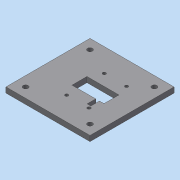
# Autodesk Inventor part: Part2
Saved by Autodesk Inventor 2016 SP1 (Build 200210100, 210)
## iProperties
Created: 2016-03-20
Part Number: Part2
Material: Generic
Document SubType Name: Modeling
Designer: Mohamed A.
Density: 1 g/cm^3
Appearance: Default
Author: Mohamed A.
Autodesk Inventor part; units mm, degrees
ref_plane "YZ Plane" through (0, 0, 0) normal (1, 0, 0) x (0, 1, 0)
ref_plane "XZ Plane" through (0, 0, 0) normal (0, 1, 0) x (-1, 0, 0)
ref_plane "XY Plane" through (0, 0, 0) normal (0, 0, 1) x (1, 0, 0)
sketch "Sketch1" plane through (0, 0, 0) normal (0, 0, 1) x (1, 0, 0)
  line L0 (8.35, -7) -> (8.35, -9) construction
  line L1 (8.35, -9) -> (7.35, -9) construction
  line L2 (7.35, -9) -> (7.35, -7) construction
  line L3 (7.35, -7) -> (8.35, -7) construction
  line L4 (9.45, -5.5) -> (9.45, -7.5) construction
  line L5 (9.45, -7.5) -> (8.45, -7.5) construction
  line L6 (8.45, -7.5) -> (8.45, -5.5) construction
  line L7 (8.45, -5.5) -> (9.45, -5.5) construction
  line L8 (2.45, 4.2) -> (2.45, -4.2) construction
  line L9 (2.45, -4.2) -> (-5.95, -4.2) construction
  line L10 (-5.95, -4.2) -> (-5.95, 4.2) construction
  line L11 (-5.95, 4.2) -> (2.45, 4.2) construction
  circle A0 centre (-2.6, 10.5) radius 1 construction
  circle A1 centre (9.9, 10.5) radius 1 construction
  circle A2 centre (-2.6, -10.5) radius 1 construction
  circle A3 centre (9.9, -10.5) radius 1 construction
  line L12 (11.95, 12.5) -> (-11.95, 12.5) projected
  line L13 (-11.95, 12.5) -> (-11.95, -12.5) projected
  line L14 (-11.95, -12.5) -> (11.95, -12.5) projected
  line L15 (11.95, -12.5) -> (11.95, 12.5) construction
  line L16 (5.7177, -12.5) -> (14.5315, -12.5) construction
  line L17 (11.95, -4.2) -> (9.45, -4.2)
  line L18 (-5.95, -4.2) -> (-5.95, 4.2)
  line L19 (-5.95, 4.2) -> (11.95, 4.2)
  line L20 (7.35, -4.2) -> (7.35, -9)
  line L21 (7.35, -9) -> (9.45, -9)
  line L22 (9.45, -9) -> (9.45, -4.2)
  line L23 (7.35, -4.2) -> (-5.95, -4.2)
  circle A4 centre (-2.6, -10.5) radius 0.9
  circle A5 centre (9.9, -10.5) radius 0.9
  circle A6 centre (9.9, 10.5) radius 0.9
  circle A7 centre (-2.6, 10.5) radius 0.9
  line L24 (23.45, 23.5) -> (23.45, -23.5) projected
  line L25 (-23.55, 23.5) -> (23.45, 23.5) projected
  line L26 (-23.55, 12.5) -> (-23.55, 23.5) projected
  line L27 (-23.55, 12.5) -> (-11.95, 12.5)
  line L28 (-11.95, -12.5) -> (-23.55, -12.5)
  line L29 (-23.55, -23.5) -> (-23.55, -12.5) projected
  line L30 (23.45, -23.5) -> (-23.55, -23.5) projected
  line L31 (11.95, 4.2) -> (11.95, -4.2)
  line L32 (-23.55, 12.5) -> (-23.55, -12.5)
  circle A8 centre (-18.05, 18) radius 1.4 projected
  circle A9 centre (17.95, 18) radius 1.4 projected
  circle A10 centre (17.95, -18) radius 1.4 projected
  circle A11 centre (-18.05, -18) radius 1.4 projected
  point P0 (0, 0)
  dimension "d4" = 1.8
  dimension "d5" = 1.8
  dimension "d6" = 1.8
  dimension "d7" = 1.8
  constraints: 24 end point, 4 centre point, 4 coincident, 4 collinear, 4 horizontal, 4 perpendicular, 4 point on line, 2 vertical
  measures "d4" diameter of A4
  measures "d5" diameter of A5
  measures "d6" diameter of A6
  measures "d7" diameter of A7
extrude "Extrusion1" add sketch "Sketch1" along normal blind 3
body "Solid1"
